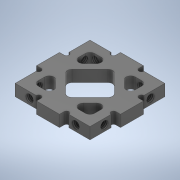
# Autodesk Inventor part: UpperArm_diagonal
Saved by Autodesk Inventor 2020.4 (Build 244396000, 396)
## iProperties
Part Number: UpperArm_diagonal
Material: アセタール樹脂、黒
Document SubType Name: Modeling
Designer: Masato Kubotera
Density: 1.425 g/cm^3
Appearance: 滑らか - 黒
Description: POM T5
Mass: 5.01849 g
Surface Area: 32.301 cm^2
Volume: 3.52175 cm^3
Author: Masato Kubotera
Autodesk Inventor part; units mm, degrees
ref_plane "YZ Plane" through (0, 0, 0) normal (1, 0, 0) x (0, 1, 0)
ref_plane "XZ Plane" through (0, 0, 0) normal (0, 1, 0) x (-1, 0, 0)
ref_plane "XY Plane" through (0, 0, 0) normal (0, 0, 1) x (1, 0, 0)
sketch "スケッチ1" plane through (0, 0, 0) normal (0, 0, 1) x (1, 0, 0)
  line L0 (-16.25, 0) -> (0, 0) construction
  line L1 (0, 0) -> (0, 0)
  line L2 (-16.25, -16.25) -> (-16.25, 0) construction
  line L3 (0, 0) -> (-16.25, -16.25)
  line L4 (-5, -18.25) -> (0, -18.25)
  line L5 (0, -18.25) -> (0, 0)
  line L6 (-5, -18.25) -> (-5, -16.25)
  arc A0 (-5, -16.25) -> (-7.1, -16.25) centre (-6.05, -16.25) ccw
  line L7 (-16.25, -16.25) -> (-7.1, -16.25)
  line L8 (-5.3033, -5.3033) -> (0, -10.6066)
  line L9 (-12.25, -12.25) -> (-2.5992, -12.25)
  line L10 (-2.5992, -12.25) -> (-7.4246, -7.4246)
  line L11 (-12.25, -12.25) -> (-12.25, -2.5992) construction
  arc A1 (-12.25, -10.25) -> (-10.25, -12.25) centre (-10.25, -10.25) ccw
  line L12 (-10, -16.25) -> (-10, -12.25) construction
  line L13 (-8, -16.25) -> (-8, -12.25) construction
  line L14 (-12, -16.25) -> (-12, -12.25) construction
  point P0 (-11.6642, -11.6642)
  dimension "d33" = 16.25
  dimension "d34" = 16.25
  dimension "d38" = 5
  dimension "d39" = 1.05
  dimension "d40" = 3
  dimension "d41" = 4
  dimension "d42" = 7.5
  dimension "d43" = 2
  dimension "d59" = 2
  dimension "d61" = 10
  dimension "d62" = 4
  constraints: 30 end point, 15 point on line, 7 perpendicular, 4 horizontal, 4 point on circle, 2 centre point, 2 coincident, 2 symmetric about line, 2 tangent, 1 parallel, 1 vertical
  measures "d33" distance of L0.start L0.end
  measures "d34" distance of L2.start L0.start
  measures "d38" distance of L4.start L4.end
  measures "d39" radius of A0
  measures "d40" distance between parallel lines of L10 L8
  measures "d41" distance between parallel lines of L7 L9
  measures "d42" distance from line of L8 L0.end
  measures "d43" distance of L4.start L6.end
  measures "d59" radius of A1
  measures "d61" distance between parallel lines of L5 L12
  measures "d62" distance between parallel lines of L13 L14
extrude "押し出し1" add sketch "スケッチ1" along normal mid plane 5 contours L8 L5 L4 L6 A0 L7 L3 L9 L10 | A1 L9 L3
sketch "スケッチ2" plane through (-7.1, -16.25, -2.5) normal (0, -1, 0) x (1, 0, 0)
  line L0 (2.1, 5) -> (2.1, 0) projected
  line L1 (7.1, 0) -> (7.1, 5) projected
  line L2 (0, 0) -> (-9.15, 0) projected
  point P0 (-2.9, 2.5)
  dimension "d56" = 10
  dimension "d60" = 2.5
  measures "d56" distance from line of L1 point (-2.9, 2.5)
  measures "d60" distance from line of L2 point (-2.9, 2.5)
hole "穴1" at (-10, -16.25, 0) direction (0, 1, 0) diameter 3.242 depth 4 tip angle 118 thread size "M4x0.7" class "6H" standard "ISO Metric profile"
mirror "ミラー1" about plane through (0, -18.25, 0) normal (1, 0, 0) of "押し出し1", "穴1"
mirror "ミラー2" about plane through (11.6642, -11.6642, 0) normal (0.7071068, 0.7071068, 0) of "押し出し1", "穴1", "ミラー1"
mirror "ミラー3" about plane through (11.6642, 11.6642, 0) normal (-0.7071068, 0.7071068, 0) of "押し出し1", "穴1", "ミラー1", "ミラー2"
fillet "フィレット1" radius 2 12 edges at (-2.5992, -12.25, 0) (-12.25, -2.5992, 0) (0, -10.6066, 0) (-10.6066, 0, 0) (0, 10.6066, 0) (10.6066, 0, 0) (12.25, -2.5992, 0) (12.25, 2.5992, 0) (-2.5992, 12.25, 0) (-12.25, 2.5992, 0) (2.5992, -12.25, 0) (2.5992, 12.25, 0)
equation "\"d34\" = d33"
